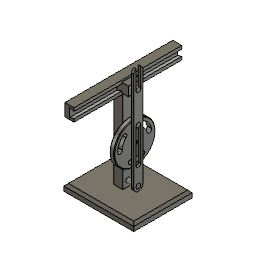
quick return mechanism (Autodesk Fusion 360 design; units mm, degrees)
part number: 2026-03-23-17-08-28-634
part number: 2026-03-23-17-18-07-780
part number: 2026-03-23-17-20-53-505
part number: 2026-03-23-17-23-14-151
part number: 2026-03-23-17-36-13-285
Autodesk Fusion 360 part; units mm, degrees
sketch "Sketch1" plane through (0, 0, 0) normal (0, 0, 1) x (1, 0, 0)
  line L0 (610, -60) -> (-610, -60)
  line L1 (-610, -60) -> (-610, 60)
  line L2 (-610, 60) -> (610, 60)
  line L3 (610, 60) -> (610, -60)
  line L4 (610, -60) -> (-610, 60) construction
  line L5 (-610, -60) -> (610, 60) construction
  line L6 (-160, 60) -> (0, 60)
  line L7 (0, 60) -> (0, 1720)
  line L8 (0, 1720) -> (-160, 1720)
  line L9 (-160, 1720) -> (-160, 60)
  line L10 (0, 0) -> (0, 60)
  line L11 (0, 160) -> (180, 160)
  line L12 (180, 160) -> (180, 200)
  line L13 (180, 200) -> (0, 200)
  line L14 (0, 200) -> (0, 160)
  line L15 (0, 780) -> (120, 780)
  line L16 (120, 780) -> (120, 820)
  line L17 (120, 820) -> (0, 820)
  line L18 (0, 820) -> (0, 780)
  line L19 (0, 1530) -> (120, 1530)
  line L20 (120, 1530) -> (120, 1690)
  line L21 (120, 1690) -> (0, 1690)
  line L22 (0, 1690) -> (0, 1530)
  line L23 (0, 1500) -> (-160, 1500)
  line L24 (0, 1610) -> (-80, 1610) construction
  line L25 (-80, 1610) -> (-80, 1690)
  line L26 (-80, 1690) -> (0, 1664.0064)
  line L27 (-80, 1530) -> (0, 1555.9936)
  line L28 (-80, 1610) -> (-80, 1530)
  line L29 (120, 1610) -> (180, 1610)
  line L30 (180, 1610) -> (180, 1650)
  line L31 (180, 1650) -> (120, 1650)
  line L32 (120, 1650) -> (120, 1610)
  line L33 (120, 820) -> (40, 820)
  line L34 (40, 820) -> (40, 1140)
  line L35 (40, 1140) -> (120, 1140)
  line L36 (120, 1140) -> (120, 820)
  line L37 (120, 1110) -> (120, 1140.0257)
  line L38 (120, 1120) -> (180, 1120)
  line L39 (180, 1120) -> (180, 1080)
  line L40 (180, 1080) -> (120, 1080)
  line L41 (120, 1080) -> (120, 1120)
  dimension "d1" = 1220
  dimension "d2" = 120
  dimension "d3" = 160
  dimension "d4" = 1660
  dimension "d5" = 100
  dimension "d6" = 40
  dimension "d7" = 720
  dimension "d8" = 40
  dimension "d9" = 30
  dimension "d10" = 160
  dimension "d11" = 120
  dimension "d12" = -220
  dimension "d13" = 80
  dimension "d14" = 18
  dimension "d15" = 40
  dimension "d16" = 320
  dimension "d17" = 80
  dimension "d18" = 20
  dimension "d19" = 40
  dimension "d20" = 60
  constraint horizontal L0
  constraint perpendicular L0 L1
  constraint parallel L0 L2
  constraint parallel L1 L3
  constraint coincident L4 L10.start
  constraint coincident L5 L10.start
  constraint coincident L10.start origin
  constraint horizontal L6
  constraint vertical L7
  constraint horizontal L8
  constraint vertical L9
  constraint midpoint L2 L6.end
  constraint coincident L6.end L7.start
  constraint horizontal L11
  constraint vertical L12
  constraint horizontal L13
  constraint vertical L14
  constraint coincident L7 L11.start
  constraint horizontal L15
  constraint vertical L16
  constraint horizontal L17
  constraint vertical L18
  constraint coincident L7 L15.start
  constraint horizontal L19
  constraint vertical L20
  constraint horizontal L21
  constraint vertical L22
  constraint coincident L7 L19.start
  constraint horizontal L24
  constraint midpoint L22 L24.start
  constraint perpendicular L24 L25
  constraint coincident L22 L26.end
  constraint horizontal L21.end L25.end
  constraint symmetric L25.start L24 L28.start
  constraint symmetric L24 L25.end L27.start
  constraint symmetric L24 L26.end L27.end
  constraint horizontal L29
  constraint vertical L30
  constraint horizontal L31
  constraint vertical L32
  constraint midpoint L20 L29.start
  constraint horizontal L33
  constraint vertical L34
  constraint horizontal L35
  constraint vertical L36
  constraint vertical L37
  constraint coincident L36 L37.end
  constraint horizontal L38
  constraint vertical L39
  constraint horizontal L40
  constraint vertical L41
  constraint coincident L36 L38.start
  constraint vertical L29.end L38.end
  constraint vertical L19.end L37.end
  constraint vertical L12.end L39.end
  measures "d1" distance of L1.end L2.end
  measures "d2" distance of L0.end L1.end
  measures "d3" distance of L6.start L6.end
  measures "d4" distance of L6.start L8.end
  measures "d5" distance of L2 L11.end
  measures "d6" distance of L11.end L12.end
  measures "d7" vertical distance of L2.end L15.end
  measures "d8" distance of L15.end L16.end
  measures "d9" vertical distance of L7.end L20.end
  measures "d10" distance of L19.end L20.end
  measures "d11" distance of L20.end L21.end
  measures "d13" distance of L24.start L24.end
  measures "d14" angle of L21 L26
  measures "d15" distance of L29.start L31.end
  measures "d16" distance of L33.end L34.end
  measures "d17" distance of L34.end L35.end
  measures "d18" vertical distance of L35.end L38.end
  measures "d19" distance of L38.end L39.end
  measures "d20" distance of L29.start L29.end
extrude "Extrude1" add sketch "Sketch1" along normal mid plane 1020 contours L0 L1 L2 L3 L6 makes body 1 in component "base"
extrude "Extrude1'" add sketch "Sketch1" along normal mid plane 1880 separate body contours L7 L8 L9 L22 L23 L25 L26 L27 L28 makes body 2
extrude "Extrude2" add sketch "Sketch1" along normal mid plane 180 contours L2 L6 L7 L9 L14 L18 L23 bodies 2
revolve "Revolve1" add sketch "Sketch1" angle 360 about axis through (0, 160, 0) along (1, 0, 0) contours L7 L11 L12 L13 L14 bodies 2
revolve "Revolve2" add sketch "Sketch1" angle 360 about axis through (0, 780, 0) along (1, 0, 0) contours L7 L15 L16 L17 L18 L33 bodies 2
extrude "Extrude1''" add sketch "Sketch1" along normal mid plane 220 separate body contours L7 L19 L20 L21 L22 L32 | L7 L22 L25 L26 L27 L28 makes body 3 in component "slider"
revolve "Revolve1'" add sketch "Sketch1" angle 360 about axis through (120, 1610, 0) along (1, 0, 0) contours L20 L29 L30 L31 L32 bodies 3 in component "slider"
revolve "Revolve1''" add sketch "Sketch1" angle 360 about axis through (120, 780, 0) along (-1, 0, 0) separate body contours L17 L33 L34 L35 L36 L37 L41 makes body 4 in component "disk"
revolve "Revolve2'" add sketch "Sketch1" angle 360 about axis through (180, 1080, 0) along (-1, 0, 0) contours L36 L37 L38 L39 L40 L41 bodies 4 in component "disk"
sketch "Sketch2" plane through (120, 0, 0) normal (1, 0, 0) x (0, 0, -1)
  circle A0 centre (0, 1080) radius 40
  circle A1 centre (0, 780) radius 360
  circle A2 centre (0, 780) radius 40
  arc A3 (-152.8248, 938.2548) -> (-220, 780) centre (0, 780) ccw
  arc A4 (-152.8248, 938.2548) -> (-208.3975, 995.8019) centre (-180.6112, 967.0283) ccw
  arc A5 (-208.3975, 995.8019) -> (-300, 780) centre (0, 780) ccw
  arc A6 (-300, 780) -> (-220, 780) centre (-260, 780) ccw
  arc A7 (-180.6112, 967.0283) -> (-260, 780) centre (0, 780) ccw construction
  line L0 (-180.6112, 967.0283) -> (0, 780) construction
  line L1 (0, 780) -> (-260, 780) construction
  line L2 (0, 780) -> (-360, 780) construction
  dimension "d34" = 46
  dimension "d35" = 40
  dimension "d36" = 260
  constraint tangent A3 A4
  constraint tangent A4 A5
  constraint tangent A5 A6
  constraint tangent A3 A6
  constraint coincident A1.centre A2.centre
  constraint coincident A4.centre A7.start
  constraint coincident A6.centre A7.end
  constraint coincident A1 L2.end
  constraint horizontal L2
  constraint coincident A6.centre L2
  measures "d34" angle of L0 L1
  measures "d35" radius of A4
  measures "d36" radius of A7
extrude "Extrude1'''" cut sketch "Sketch2" against normal blind 250 contours A3 A4 A5 A6 bodies 4 in component "disk"
pattern_circular "C-Pattern1" count 3 over 360 about axis through (120, 780, 0) along (1, 0, 0) of "Extrude1'''" in component "disk"
chamfer "Chamfer1" distance 10 angle 45 1 faces at (66.6667, 1139.5525, 17.9445) on bodies 4 in component "disk"
chamfer "Chamfer1'" distance 40 angle 45 4 edges at (0, 60, -510) (610, 60, 0) (0, 60, 510) (-610, 60, 0) on bodies 1 in component "base"
sketch "Sketch3" plane through (180, 0, 0) normal (1, 0, 0) x (0, 0, -1)
  circle A0 centre (0, 160) radius 40
  line L0 (80, 160) -> (80, 1880)
  arc A1 (80, 1880) -> (-80, 1880) centre (0, 1880) ccw
  line L1 (-80, 1880) -> (-80, 160)
  arc A2 (-80, 160) -> (80, 160) centre (0, 160) ccw
  line L2 (0, 160) -> (0, 1880) construction
  circle A3 centre (0, 780) radius 40
  circle A4 centre (0, 1080) radius 40
  circle A5 centre (0, 1610) radius 40
  line L3 (-40, 1080) -> (-40, 480)
  arc A6 (-40, 480) -> (40, 480) centre (0, 480) ccw
  line L4 (40, 480) -> (40, 1080)
  arc A7 (40, 1080) -> (-40, 1080) centre (0, 1080) ccw
  line L5 (0, 1080) -> (0, 480) construction
  line L6 (40, 1610) -> (40, 1960)
  arc A8 (40, 1960) -> (-40, 1960) centre (0, 1960) ccw
  line L7 (-40, 1960) -> (-40, 1610)
  arc A9 (-40, 1610) -> (40, 1610) centre (0, 1610) ccw
  line L8 (0, 1610) -> (0, 1960) construction
  dimension "d43" = 1720
  dimension "d44" = 80
  constraint tangent L0 A1
  constraint tangent A1 L1
  constraint parallel L0 L1
  constraint tangent L1 A2
  constraint tangent L0 A2
  constraint vertical L2
  constraint coincident A0.centre A2.centre
  constraint tangent L3 A6
  constraint tangent A6 L4
  constraint parallel L3 L4
  constraint tangent L4 A7
  constraint tangent L3 A7
  constraint coincident L2 A6.centre
  constraint parallel L2 L5
  constraint coincident A4.centre A7.centre
  constraint equal A4 A7
  constraint tangent L6 A8
  constraint tangent A8 L7
  constraint parallel L6 L7
  constraint tangent L7 A9
  constraint tangent L6 A9
  constraint parallel L0 L8
  constraint coincident A5.centre A9.centre
  constraint coincident A1 A8.centre
  measures "d43" distance of A0.centre A1.centre
  measures "d44" radius of A1
extrude "Extrude1''''" add sketch "Sketch3" against normal blind 40 separate body contours L0 A1 L1 A2 A5 L6 L7 A9 makes body 5 in component "crank"
combine "Combine1" operation add target body 1 tool bodies 2 in component "base"
component "base" placed x (1, 0, 0) y (0, 1, 0) z (0, 0, 1) at (0, 0, 0)
component "slider" placed x (1, 0, 0) y (0, 1, 0) z (0, 0, 1) at (0, 0, 0.338)
component "disk" placed x (1, 0, 0) y (0, 1, 0) z (0, 0, 1) at (0, 0, 0)
component "crank" placed x (1, 0, 0) y (0, 1, 0) z (0, 0, 1) at (0, 0, 0)
